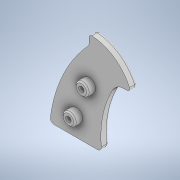
# Autodesk Inventor part: Rukohvat_Levi_2
Saved by Autodesk Inventor 2021 (Build 250183000, 183)
## iProperties
Created: 2022-03-09
Part Number: Rukohvat_Levi_2
Material: Generic
Document SubType Name: Modeling
Designer: Carlos Montoya
Density: 1 g/cm^3
Appearance: Default
Author: Carlos Montoya
Autodesk Inventor part; units mm, degrees
ref_plane "YZ Plane" through (0, 0, 0) normal (1, 0, 0) x (0, 1, 0)
ref_plane "XZ Plane" through (0, 0, 0) normal (0, 1, 0) x (-1, 0, 0)
ref_plane "XY Plane" through (0, 0, 0) normal (0, 0, 1) x (1, 0, 0)
sketch "Sketch1" plane through (0, 0, 0) normal (0, 0, 1) x (1, 0, 0)
  arc A0 (26.2029, 65.6915) -> (-2.973, 3.4018) centre (110.991, -12) ccw
  line L0 (26.991, 71.9374) -> (26.991, 67.7183)
  arc A1 (26.2029, 65.6915) -> (26.991, 67.7183) centre (23.991, 67.7183) ccw
  arc A2 (29.116, 73.9335) -> (26.991, 71.9374) centre (28.991, 71.9374) ccw
  arc A3 (58.0589, 53.8125) -> (29.116, 73.9335) centre (26.991, 40) ccw
  arc A4 (56.2314, 51) -> (58.0589, 53.8125) centre (56.2314, 53) ccw
  line L1 (53.8596, 51) -> (56.2314, 51)
  arc A5 (53.8596, 51) -> (45.0701, 45.7692) centre (53.8596, 41) ccw
  arc A6 (45.0701, 45.7692) -> (36.2936, 3.2692) centre (110.991, 10) ccw
  arc A7 (33.3057, 0) -> (36.2936, 3.2692) centre (33.3057, 3) ccw
  line L2 (0, 0) -> (33.3057, 0)
  arc A8 (-2.973, 3.4018) -> (0, 0) centre (0, 3) ccw
  constraints: 18 point on circle, 9 centre point, 6 end point
extrude "Extrusion1" add sketch "Sketch1" along normal blind 6
fillet "Fillet1" radius 2 12 edges at (57.9084, 51.9103, 0) (46.3986, 67.9167, 0) (27.6217, 73.3952, 0) (26.991, 69.8278, 0) (26.787, 66.631, 0) (6.8488, 36.7791, 0) (-2.2589, 1.0258, 0) (16.6529, 0, 0) (35.5202, 0.9761, 0) (37.5408, 25.1679, 0) (48.7455, 49.5934, 0) (55.0455, 51, 0)
sketch "Sketch2" plane through (0, 0, 6) normal (0, 0, 1) x (1, 0, 0)
  circle A0 centre (16.991, 15) radius 5
  circle A1 centre (26.991, 40) radius 5
  circle A2 centre (16.991, 15) radius 2.1
  circle A3 centre (26.991, 40) radius 2.1
  point P0 (0, 0)
  constraints: 4 centre point
extrude "Extrusion2" add sketch "Sketch2" along normal blind 6
chamfer "Chamfer1" distance 1 angle 45 2 edges at (21.991, 40, 12) (11.991, 15, 12)
chamfer "Chamfer2" distance 2 angle 45 1 edges at (24.891, 40, 6)
chamfer "Chamfer3" distance 2 angle 45 1 edges at (14.891, 15, 6)
body "Solid1"
